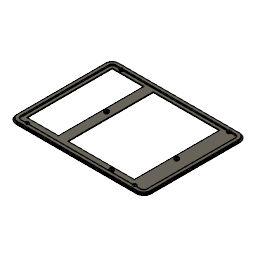
Mini PC Lid V1 (Autodesk Fusion 360 design; units mm, degrees)
Autodesk Fusion 360 part; units mm, degrees
sketch "Sketch1" plane through (0, 0, 0) normal (0, 0, 1) x (1, 0, 0)
  line L0 (10, 0) -> (200, 0)
  line L1 (210, 10) -> (210, 150)
  line L2 (200, 160) -> (10, 160)
  line L3 (0, 150) -> (0, 10)
  arc A0 (10, 160) -> (0, 150) centre (10, 150) ccw
  arc A1 (210, 150) -> (200, 160) centre (200, 150) ccw
  arc A2 (200, 0) -> (210, 10) centre (200, 10) ccw
  arc A3 (0, 10) -> (10, 0) centre (10, 10) ccw
  line L4 (200, 162) -> (10, 162)
  arc A4 (10, 162) -> (-2, 150) centre (10, 150) ccw
  line L5 (-2, 150) -> (-2, 10)
  arc A5 (-2, 10) -> (10, -2) centre (10, 10) ccw
  line L6 (10, -2) -> (200, -2)
  arc A6 (200, -2) -> (212, 10) centre (200, 10) ccw
  line L7 (212, 10) -> (212, 150)
  arc A7 (212, 150) -> (200, 162) centre (200, 150) ccw
  line L8 (200, 155) -> (10, 155)
  arc A8 (10, 155) -> (5, 150) centre (10, 150) ccw
  line L9 (5, 150) -> (5, 10)
  arc A9 (5, 10) -> (10, 5) centre (10, 10) ccw
  line L10 (10, 5) -> (200, 5)
  arc A10 (200, 5) -> (205, 10) centre (200, 10) ccw
  line L11 (205, 10) -> (205, 150)
  arc A11 (205, 150) -> (200, 155) centre (200, 150) ccw
  circle A12 centre (20, 5) radius 1.1
  circle A13 centre (20, 5) radius 3
  circle A14 centre (66, 85) radius 1.1
  circle A15 centre (186, 76) radius 1.1
  circle A16 centre (150, 9) radius 1.1
  circle A17 centre (150, 9) radius 3
  circle A18 centre (66, 85) radius 3
  circle A19 centre (186, 76) radius 3
  line L12 (105, 162) -> (105, -2) construction
  line L13 (212, 80) -> (-2, 80) construction
  circle A20 centre (190, 5) radius 3
  circle A21 centre (190, 5) radius 1.1
  circle A22 centre (20, 155) radius 3
  circle A23 centre (20, 155) radius 1.1
  circle A24 centre (190, 155) radius 3
  circle A25 centre (190, 155) radius 1.1
  point P0 (210, 0)
  point P1 (0, 160)
  dimension "d1" = 210
  dimension "d2" = 160
  dimension "d4" = 10
  dimension "d5" = 2
  dimension "d6" = -5
  dimension "d9" = 2.2
  dimension "d10" = 6
  dimension "d11" = 20
  dimension "d12" = 5
  dimension "d13" = 2.2
  dimension "d14" = 2.2
  dimension "d15" = 2.2
  dimension "d17" = 75
  dimension "d18" = 84
  dimension "d19" = 24
  dimension "d21" = 60
  dimension "d22" = 9
  dimension "d23" = 66
  dimension "d24" = 6
  dimension "d25" = 6
  dimension "d26" = 6
  dimension "d31" = 170
  dimension "d32" = 150
  constraint horizontal L0
  constraint vertical L1
  constraint horizontal L2
  constraint vertical L3
  constraint coincident P1 L2
  constraint coincident P1 L3
  constraint tangent L2 A0
  constraint tangent L3 A0
  constraint tangent L1 A1
  constraint tangent L2 A1
  constraint equal A0 A1
  constraint coincident P0 L0
  constraint coincident P0 L1
  constraint tangent L0 A2
  constraint tangent L1 A2
  constraint equal A0 A2
  constraint coincident origin L0
  constraint coincident origin L3
  constraint tangent L0 A3
  constraint tangent L3 A3
  constraint equal A0 A3
  constraint concentric A12 A13
  constraint concentric A16 A17
  constraint concentric A14 A18
  constraint concentric A15 A19
  constraint midpoint L4 L12.start
  constraint midpoint L6 L12.end
  constraint midpoint L7 L13.start
  constraint midpoint L5 L13.end
  measures "d1" distance of origin P0
  measures "d2" distance of origin P1
  measures "d4" radius of A0
  measures "d9" diameter of A12
  measures "d10" diameter of A13
  measures "d11" distance of L3 A12.centre
  measures "d12" distance of L0 A12.centre
  measures "d13" diameter of A14
  measures "d14" diameter of A15
  measures "d15" diameter of A16
  measures "d17" distance of L2 A14.centre
  measures "d18" distance of L2 A15.centre
  measures "d19" distance of L1 A15.centre
  measures "d21" distance of L1 A16.centre
  measures "d22" distance of L0 A16.centre
  measures "d23" distance of L3 A14.centre
  measures "d24" diameter of A17
  measures "d25" diameter of A18
  measures "d26" diameter of A19
extrude "Extrude1" add sketch "Sketch1" against normal blind 1 contours L0 L1 L2 L3 A0 A1 A2 A3 | L4 A4 L5 A5 L6 A6 L7 A7 | L8 A8 L9 A9 L10 A10 L11 A11 A13 A20 A22 A24 | L8 A24 A25 | L8 A24 A25 | L8 A25 | L8 A25 | L8 A22 A23 | L8 A22 A23 | L8 A23 | L8 A23 | L10 A20 A21 | L10 A20 A21 | L10 A21 | L10 A21 | L10 A12 A13 | L10 A12 A13 | L10 A12 | L10 A12 | A14 | A15 | A16 | A17 | A18 | A19
extrude "Extrude2" add sketch "Sketch1" along normal blind 2 contours L0 L1 L2 L3 A0 A1 A2 A3 | L8 A24 A25 | L8 A24 A25 | L8 A22 A23 | L8 A22 A23 | L10 A20 A21 | L10 A20 A21 | L10 A12 A13 | L10 A12 A13 | A17 | A18 | A19
sketch "Sketch2" plane through (0, 0, 0) normal (0, 0, 1) x (1, 0, 0)
  line L0 (75, 150) -> (180, 150)
  line L1 (180, 150) -> (180, 15)
  line L2 (180, 15) -> (75, 15)
  line L3 (75, 15) -> (75, 150)
  line L4 (60, 15) -> (10, 15)
  line L5 (10, 15) -> (10, 150)
  line L6 (10, 150) -> (60, 150)
  line L7 (60, 150) -> (60, 15)
  constraint horizontal L0
  constraint vertical L1
  constraint horizontal L2
  constraint vertical L3
  constraint horizontal L4
  constraint vertical L5
  constraint horizontal L6
  constraint vertical L7
extrude "Extrude3" cut sketch "Sketch2" sketch "Sketch1" 2 faces at (66.134, 84.6587, 0) (20.2888, 5.3004, 0) against normal blind 1 of sketch 2 contours L8 A25 | L8 A25 | L8 A23 | L8 A23 | L10 A21 | L10 A21 | L10 A12 | A15 | A16 picked at (20.301, 5.4631)
sketch "Sketch3" plane through (0, 0, -1) normal (0, 0, -1) x (1, 0, 0)
  circle A0 centre (66, -85) radius 1.1
  circle A1 centre (150, -9) radius 1.1
  circle A2 centre (20, -155) radius 1.1
  circle A3 centre (186, -76) radius 1.1
  line L0 (180, -15) -> (180, -150)
  line L1 (180, -150) -> (75, -150)
  line L2 (75, -150) -> (75, -15)
  line L3 (75, -15) -> (180, -15)
  line L4 (10, -150) -> (10, -15)
  line L5 (10, -15) -> (60, -15)
  line L6 (60, -15) -> (60, -150)
  line L7 (60, -150) -> (10, -150)
  circle A4 centre (190, -5) radius 1.1
  circle A5 centre (190, -155) radius 1.1
  circle A6 centre (20, -5) radius 1.1
  arc A7 (200, -162) -> (212, -150) centre (200, -150) ccw
  line L8 (212, -150) -> (212, -10)
  arc A8 (212, -10) -> (200, 2) centre (200, -10) ccw
  line L9 (200, 2) -> (10, 2)
  arc A9 (10, 2) -> (-2, -10) centre (10, -10) ccw
  line L10 (-2, -10) -> (-2, -150)
  arc A10 (-2, -150) -> (10, -162) centre (10, -150) ccw
  line L11 (10, -162) -> (200, -162)
  circle A11 centre (190, -155) radius 2.25
  circle A12 centre (20, -155) radius 2.25
  circle A13 centre (66, -85) radius 2.25
  circle A14 centre (186, -76) radius 2.25
  circle A15 centre (190, -5) radius 2.25
  circle A16 centre (150, -9) radius 2.25
  circle A17 centre (20, -5) radius 2.25
  dimension "d38" = 4.5
  dimension "d39" = 4.5
  dimension "d40" = 4.5
  dimension "d41" = 4.5
  dimension "d42" = 4.5
  dimension "d43" = 4.5
  dimension "d44" = 4.5
  constraint concentric A5 A11
  constraint concentric A2 A12
  constraint concentric A0 A13
  constraint concentric A3 A14
  constraint concentric A4 A15
  constraint concentric A1 A16
  constraint concentric A6 A17
  measures "d38" diameter of A11
  measures "d39" diameter of A12
  measures "d40" diameter of A13
  measures "d41" diameter of A14
  measures "d42" diameter of A15
  measures "d43" diameter of A16
  measures "d44" diameter of A17
extrude "Extrude4" cut sketch "Sketch3" against normal blind 2 contours A11 | A12 | A13 | A14 | A15 | A16 | A17
equation "BoxRadius = 10 mm"
equation "d4 = BoxRadius"
equation "HolesRadius = 2.2 mm"
equation "HolesOuterRadius = 6 mm"
equation "d9 = HolesRadius"
equation "d10 = HolesOuterRadius"
equation "d13 = HolesRadius"
equation "d14 = HolesRadius"
equation "d15 = HolesRadius"
equation "d24 = HolesOuterRadius"
equation "d25 = HolesOuterRadius"
equation "d26 = HolesOuterRadius"
equation "BoltHead = 4.5 mm"
equation "d38 = BoltHead"
equation "d39 = BoltHead"
equation "d40 = BoltHead"
equation "d41 = BoltHead"
equation "d42 = BoltHead"
equation "d43 = BoltHead"
equation "d44 = BoltHead"
